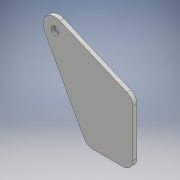
# Autodesk Inventor part: flange_large
Saved by Autodesk Inventor 2017 (Build 210142000, 142)
## iProperties
Created: 2016-09-16
Part Number: flange_large
Material: Generic
Document SubType Name: Modeling
Designer: Nic
Density: 1 g/cm^3
Appearance: Default
Author: Nic
Autodesk Inventor part; units mm, degrees
ref_plane "YZ Plane" through (0, 0, 0) normal (1, 0, 0) x (0, 1, 0)
ref_plane "XZ Plane" through (0, 0, 0) normal (0, 1, 0) x (-1, 0, 0)
ref_plane "XY Plane" through (0, 0, 0) normal (0, 0, 1) x (1, 0, 0)
sketch "Sketch1" plane through (0, 0, 0) normal (0, 1, 0) x (-1, 0, 0)
  circle A0 centre (0, 0) radius 12 construction
  line L0 (0, 0) -> (0, -50) construction
  line L1 (-20, -16) -> (-34, -16) construction
  line L2 (-34, -16) -> (-34, -50) construction
  line L3 (-34, -50) -> (-20, -50) construction
  line L4 (-20, -50) -> (-20, -16) construction
  circle A1 centre (0, 0) radius 2
  arc A2 (5.2716, -2.8654) -> (-2.3397, 5.525) centre (0, 0) ccw
  line L5 (-34, -42) -> (-18.9731, -42)
  line L6 (5.2716, -2.8654) -> (-14.5801, -39.3878)
  line L7 (-2.3397, 5.525) -> (-35.9498, -8.7083)
  line L8 (-39, -13.3125) -> (-39, -37)
  arc A3 (-18.9731, -42) -> (-14.5801, -39.3878) centre (-18.9731, -37) ccw
  arc A4 (-39, -37) -> (-34, -42) centre (-34, -37) ccw
  arc A5 (-35.9498, -8.7083) -> (-39, -13.3125) centre (-34, -13.3125) ccw
  point P0 (-39, -42)
  point P1 (-16, -42)
  point P2 (-39, -10)
  dimension "d0" = 50
  dimension "d1" = 24
  dimension "d2" = 14
  dimension "d3" = 34
  dimension "d4" = 16
  dimension "d5" = 20
  dimension "d6" = 4
  dimension "d7" = 12
  dimension "d8" = 26
  dimension "d9" = 23
  dimension "d10" = 5
  dimension "d11" = 32
  dimension "d12" = 5
  dimension "d13" = 5
  constraints: 18 end point, 8 point on circle, 8 tangent, 6 centre point, 6 point on line, 3 coincident, 2 horizontal, 2 parallel, 2 vertical, 1 equal radius, 1 perpendicular
  measures "d0" distance of L0.start L0.end
  measures "d1" diameter of A0
  measures "d2" distance between parallel lines of L2 L4
  measures "d3" distance of L1.end L2.end
  measures "d4" distance from line of point (0, 0) L1
  measures "d5" distance from line of point (0, 0) L4
  measures "d6" diameter of A1
  measures "d7" diameter of A2
  measures "d8" distance between parallel lines of L1 L5
  measures "d9" distance of point (-39, -42) point (-16, -42)
  measures "d10" distance between parallel lines of L2 L8
  measures "d11" distance of point (-39, -10) point (-39, -42)
  measures "d12" radius of A3
  measures "d13" radius of A4
extrude "Extrusion1" add sketch "Sketch1" along normal blind 2
body "Solid1"
